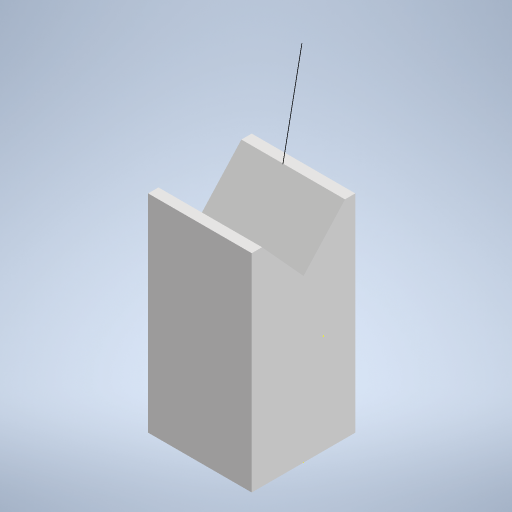
# Autodesk Inventor part: хвост
Saved by Autodesk Inventor 2024.2 (Build 282272000, 272)
## iProperties
Created: 2026-04-03
Part Number: хвост
Material: Типовые
Document SubType Name: Modeling
Designer: katya_notebook
Density: 1 g/cm^3
Appearance: По умолчанию
Author: katya_notebook
Autodesk Inventor part; units mm, degrees
ref_plane "YZ Plane" through (0, 0, 0) normal (1, 0, 0) x (0, 1, 0)
ref_plane "XZ Plane" through (0, 0, 0) normal (0, 1, 0) x (-1, 0, 0)
ref_plane "XY Plane" through (0, 0, 0) normal (0, 0, 1) x (1, 0, 0)
sketch "Эскиз4" plane through (0, 0, 0) normal (1, 0, 0) x (0, 1, 0)
  line L0 (-40, -20) -> (40, -20)
  line L1 (40, -20) -> (40, 20)
  line L2 (40, 20) -> (-40, 20)
  line L3 (-40, 20) -> (-40, -20)
  line L4 (-40, -20) -> (40, 20) construction
  line L5 (40, -20) -> (-40, 20) construction
  line L6 (22.4045, 0) -> (40, 16)
  line L7 (40, 16) -> (-40, 0)
  line L8 (22.4045, 0) -> (40, -16)
  line L9 (-40, 0) -> (40, -16)
  line L10 (0, 0) -> (40, 0)
  dimension "d2" = 80
  dimension "d3" = 40
  dimension "d4" = 16
  dimension "d5" = 16
  constraints: 22 end point, 4 midpoint, 3 point on line, 2 parallel, 1 horizontal, 1 perpendicular
  measures "d2" distance of L1.end L2.end
  measures "d3" distance of L0.end L1.end
  measures "d4" vertical distance of L6.start L8.end
  measures "d5" vertical distance of L6.end L6.start
extrude "Выдавливание1" add sketch "Эскиз4" against normal blind 40 contours L3 L9 L1 L0 | L3 L2 L1 L7 | L7 L6 L8 L9
sketch "Эскиз5" plane through (0, -40, 0) normal (0, -0.1961161, -0.9805807) x (-1, 0, 0)
  line L0 (40, 81.5843) -> (40, 0) projected
  line L1 (34.6935, 34.7538) -> (24, 0)
  line L2 (0, 0) -> (40, 0) projected
  line L3 (40, 70.0441) -> (40, 81.5843)
  arc A0 (34.6935, 34.7538) -> (40, 70.0441) centre (-80, 70.0441) ccw
  point P0 (0, 39.2232)
  point P1 (40, 52)
  point P2 (40, 70.0441)
  dimension "d8" = 16
  dimension "d9" = 52
  dimension "d12" = 120
  constraints: 4 end point, 4 point on line, 2 point on circle, 2 tangent, 1 centre point, 1 collinear
  measures "d8" distance of L0.end L1.end
  measures "d9" distance of L0.end point (40, 52)
  measures "d12" radius of A0
extrude "Выдавливание2" [suppressed]
sketch "Эскиз6" plane through (0, 40, -16) normal (0, -0.1961161, -0.9805807) x (-1, 0, 0)
  line L0 (0, -81.5843) -> (40, -81.5843) projected
  line L1 (24, -81.5843) -> (24, 37.2051)
  point P0 (0, -42.3611)
  constraints: 2 end point, 1 vertical
sketch "Эскиз8" plane through (0, -40, -20) normal (0, -1, 0) x (1, 0, 0)
  line L0 (-40, 20) -> (-40, 4) projected
  line L1 (0, 0) -> (-40, 20)
  line L2 (0, 40) -> (0, 0) projected
  line L3 (-40, 20) -> (0, 40)
  line L4 (0, 40) -> (0, 0)
  line L5 (0, 0) -> (-40, 0)
  line L6 (-40, 0) -> (-40, 40)
  line L7 (-40, 40) -> (0, 40)
  point P0 (0, 20)
  constraints: 12 end point, 2 perpendicular, 1 collinear, 1 horizontal
extrude "Выдавливание3" [suppressed]
pattern_circular "Круговой массив2" [suppressed]
